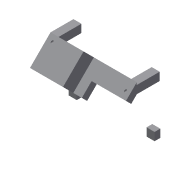
# Autodesk Inventor part: 30_CUBE_openSIM_DLP200EVM_Holder
Saved by Autodesk Inventor 2019 (Build 230136000, 136)
## iProperties
Created: 2019-08-02
Part Number: 30_CUBE_openSIM_DLP200EVM_Holder
Material: Generic
Document SubType Name: Modeling
Designer: diederichbenedict
Density: 1 g/cm^3
Appearance: Default
Author: diederichbenedict
Autodesk Inventor part; units mm, degrees
ref_plane "YZ Plane" through (0, 0, 0) normal (1, 0, 0) x (0, 1, 0)
ref_plane "XZ Plane" through (0, 0, 0) normal (0, 1, 0) x (-1, 0, 0)
ref_plane "XY Plane" through (0, 0, 0) normal (0, 0, 1) x (1, 0, 0)
ref_plane "Work Plane1" through (-61.5, 6.5, -4.5) normal (0, 0, 1) x (1, 0, 0)
sketch "Sketch1" plane through (-61.5, 6.5, -4.5) normal (0, 0, 1) x (1, 0, 0)
  circle A0 centre (0, 0) radius 1.7 construction
  circle A1 centre (66.5, -2.5) radius 1.1 construction
  circle A2 centre (66.5, -45.5) radius 1.1 construction
  circle A3 centre (0.5, -48) radius 1.7 construction
  line L0 (70.5084, 1.2598) -> (63.5084, 1.2598)
  line L1 (63.5084, 1.2598) -> (63.5084, -5.7402)
  line L2 (63.5084, -5.7402) -> (70.5084, -5.7402)
  line L3 (70.5084, -5.7402) -> (70.5084, 1.2598)
  circle A4 centre (68.0875, -0.9125) radius 1.1 construction
  line L4 (70.9947, -41.5157) -> (63.9947, -41.5157)
  line L5 (63.9947, -41.5157) -> (63.9947, -48.5157)
  line L6 (63.9947, -48.5157) -> (70.9947, -48.5157)
  line L7 (70.9947, -48.5157) -> (70.9947, -41.5157)
  circle A5 centre (69.675, 0.675) radius 1.1 construction
  line L8 (3.0987, -44.4) -> (-3.9013, -44.4)
  line L9 (-3.9013, -44.4) -> (-3.9013, -51.4)
  line L10 (-3.9013, -51.4) -> (3.0987, -51.4)
  line L11 (3.0987, -51.4) -> (3.0987, -44.4)
  circle A6 centre (71.2625, 2.2625) radius 1.1 construction
  line L12 (2.2, 3.3625) -> (-4.8, 3.3625)
  line L13 (-4.8, 3.3625) -> (-4.8, -3.6375)
  line L14 (-4.8, -3.6375) -> (2.2, -3.6375)
  line L15 (2.2, -3.6375) -> (2.2, 3.3625)
  point P0 (61.5, -6.5)
  point P1 (63.0875, -4.9125)
  point P2 (64.675, -3.325)
  point P3 (66.2625, -1.7375)
  dimension "d4" = 7
  dimension "d5" = 7
  dimension "d6" = 7
  dimension "d7" = 7
  dimension "d8" = 7
  dimension "d9" = 7
  dimension "d10" = 7
  dimension "d11" = 7
  constraints: 32 end point, 8 parallel, 4 horizontal, 4 perpendicular, 3 centre point
  measures "d4" distance of L2.end L1.end
  measures "d5" distance of L1.end L0.end
  measures "d6" distance of L6.end L5.end
  measures "d7" distance of L5.end L5.start
  measures "d8" distance of L10.end L9.end
  measures "d9" distance of L9.end L9.start
  measures "d10" distance of L14.end L13.end
  measures "d11" distance of L13.end L13.start
extrude "Extrusion1" add sketch "Sketch1" along normal blind 5
sketch "Sketch2" plane through (-61.5, 6.5, 0.5) normal (0, 0, 1) x (1, 0, 0)
  line L0 (70.5084, 1.2598) -> (63.5084, 1.2598) projected
  line L1 (63.5084, 1.2598) -> (63.5084, -5.7402) projected
  line L2 (63.5084, -5.7402) -> (70.5084, -5.7402) projected
  line L3 (70.5084, -5.7402) -> (70.5084, 1.2598) projected
  line L4 (-4.8, 3.3625) -> (-4.8, -3.6375) projected
  line L5 (-4.8, -3.6375) -> (2.2, -3.6375) projected
  line L6 (2.2, -3.6375) -> (2.2, 3.3625) projected
  line L7 (2.2, 3.3625) -> (-4.8, 3.3625) projected
  point P0 (61.5, -6.5)
extrude "Extrusion2" add sketch "Sketch2" along normal blind 15
sketch "Sketch3" plane through (-66.3, 2.8625, -4.5) normal (-1, 0, 0) x (0, 0, 1)
  line L0 (0, 4.8973) -> (0, -2.1027) projected
  line L1 (0, -2.1027) -> (20, -2.1027) projected
  line L2 (20, 4.8973) -> (20, -2.1027) projected
  line L3 (0, 4.8973) -> (20, 4.8973) projected
  line L4 (0, 0) -> (0, 7) projected
  line L5 (0, 0) -> (20, 0) projected
  line L6 (20, 7) -> (20, 0) projected
  line L7 (0, 7) -> (20, 7) projected
  line L8 (0, -2.1027) -> (20, -2.1027) projected
  line L9 (20, -2.1027) -> (20, 7)
  line L10 (0, 7) -> (20, 7) projected
  line L11 (20, 7) -> (24.5513, 2.4487)
  line L12 (20, 7) -> (26.4366, 7) construction
  line L13 (24.5513, 2.4487) -> (20, -2.1027)
  line L14 (7.5, -41.3758) -> (74.2482, 25.3723) construction
  line L15 (24.5513, 2.4487) -> (20, -2.1027)
  line L16 (20, -2.1027) -> (33.3866, -15.4893)
  line L17 (33.3866, -15.4893) -> (37.9379, -10.9379)
  line L18 (37.9379, -10.9379) -> (24.5513, 2.4487)
  point P0 (4.5, -2.8625)
  dimension "d16" = 45
  constraints: 16 end point, 4 equal length, 3 perpendicular, 1 horizontal
  measures "d16" angle of L11 L12
extrude "Extrusion3" add sketch "Sketch3" against normal up to surface (75.3084 mm away) contours L6 L11 L13 L2 | L13 L18 L17 L16
sketch "Sketch4" plane through (-61.5, 6.5, -4.5) normal (0, 0, -1) x (-1, 0, 0)
  circle A0 centre (-66.5, -2.5) radius 1.1 projected
  circle A1 centre (0, 0) radius 1.1 projected
  point P0 (-61.5, -6.5)
hole "Hole1" at (5, 4, -4.5) at (-61.5, 6.5, -4.5) direction (0, 0, 1) diameter 1.9 end through all
sketch "Sketch5" plane through (-66.3, -8.0754, 33.4379) normal (0, 0.7071068, 0.7071068) x (1, 0, 0)
  line L0 (31.8, 0) -> (67.6266, 0) projected
  line L1 (75.3084, 25.3681) -> (75.3084, 0) projected
  line L2 (75.3084, 0) -> (45.3084, 0)
  line L3 (45.3084, 0) -> (45.3084, 12)
  line L4 (45.3084, 12) -> (75.3084, 12)
  line L5 (75.3084, 12) -> (75.3084, 0)
  point P0 (66.3, 29.3544)
  dimension "d28" = 30
  dimension "d29" = 12
  constraints: 8 end point, 2 parallel, 1 horizontal, 1 perpendicular
  measures "d28" distance of L3.end L4.end
  measures "d29" distance of L2.end L3.end
extrude "Extrusion5" cut sketch "Sketch5" against normal up to surface (6.4366 mm away)
sketch "Sketch6" plane through (-66.3, -8.0754, 33.4379) normal (0, -0.7071068, 0.7071068) x (1, 0, 0)
  line L0 (45.3084, -6.4366) -> (45.3084, 0) projected
  line L1 (0, 0) -> (45.3084, 0) projected
  line L2 (0, -6.4366) -> (0, 0) projected
  line L3 (0, -6.4366) -> (45.3084, -6.4366) projected
  circle A0 centre (34.6, 8.3505) radius 1.6 projected
  circle A1 centre (34.6, -1.6495) radius 1.6 projected
  line L4 (29.8, -43.0457) -> (29.8, 51.3505) construction
  line L5 (37.8, 3.4505) -> (37.8, -42.9495) construction
  line L6 (0, -6.4366) -> (45.3084, -6.4366) construction
  line L7 (29.8, -6.4366) -> (37.8, -6.4366) construction
  line L8 (37.8, -6.4366) -> (37.8, 12.6655) construction
  line L9 (37.8, 12.6655) -> (29.8, 12.6655) construction
  line L10 (29.8, 12.6655) -> (29.8, -6.4366) construction
  line L11 (29.8, -6.4366) -> (37.8, -6.4366)
  line L12 (37.8, -6.4366) -> (37.8, 12.6655)
  line L13 (37.8, 12.6655) -> (29.8, 12.6655)
  line L14 (29.8, 12.6655) -> (29.8, -6.4366)
  point P0 (66.3, -17.934)
  constraints: 16 end point, 4 parallel, 2 horizontal, 2 perpendicular, 2 point on line
extrude "Extrusion6" add sketch "Sketch6" against normal up to surface (25.3681 mm away) contours L3 L14 L1 L12 | L1 L14 L13 L12 | A0 | A1
sketch "Sketch7" plane through (-66.3, -12.6268, 28.8866) normal (0, -0.7071068, 0.7071068) x (1, 0, 0)
  circle A0 centre (34.8, 4.987) radius 2.65 projected
  circle A1 centre (34.8, 14.987) radius 2.65 projected
  point P0 (66.3, -11.4974)
hole "Hole2" at (-31.5, -9.1004, 32.413) at (-31.5, -2.0293, 39.484) direction (0, 0.7071068, -0.7071068) diameter 2.9 end through all
body "Solid1"
